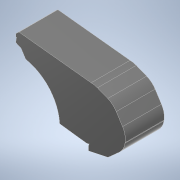
# Autodesk Inventor part: Pieza3_Carcasa
Saved by Autodesk Inventor 2022 (Build 260153000, 153)
## iProperties
Created: 2022-11-06
Part Number: Pieza3_Carcasa
Material: Resina acetálica, negra
Document SubType Name: Modeling
Designer: Mauricio Guerrero
Density: 1.425 g/cm^3
Appearance: Suave - Negro
Author: Mauricio Guerrero
## iProperties of the stored document Pieza3_Carcasa_3DPrint.ipt
Created: 2022-11-09
Part Number: Pieza3_Carcasa_3DPrint
Material: Genérico
Document SubType Name: Modeling
Designer: Mauricio Guerrero
Density: 1 g/cm^3
Appearance: Valor por defecto
Author: Mauricio Guerrero
Autodesk Inventor part; units mm, degrees
ref_plane "YZ Plane" through (0, 0, 0) normal (1, 0, 0) x (0, 1, 0)
ref_plane "XZ Plane" through (0, 0, 0) normal (0, 1, 0) x (-1, 0, 0)
ref_plane "XY Plane" through (0, 0, 0) normal (0, 0, 1) x (1, 0, 0)
sketch "Boceto1" plane through (0, 0, 0) normal (0, 0, 1) x (1, 0, 0)
  line L0 (8.9411, -4.2344) -> (11.6298, -3.6616)
  line L1 (11.6298, -3.6616) -> (13.3209, -2.1424)
  arc A0 (13.3209, -2.1424) -> (13.9587, -0.9739) centre (11.9843, -0.6546) ccw
  line L2 (13.9587, -0.9739) -> (13.978, -0.8543)
  arc A1 (9.9548, 3.6595) -> (9.2184, 3.8) centre (9.2184, 1.8) ccw
  line L3 (9.9548, 3.6595) -> (11.6833, 2.9749)
  arc A2 (12.6312, 2.1939) -> (11.6833, 2.9749) centre (10.9469, 1.1154) ccw
  line L4 (12.6312, 2.1939) -> (13.688, 0.5435)
  line L5 (14.1, 2.7373) -> (14.1, -1.982) construction
  arc A3 (13.978, -0.8543) -> (13.688, 0.5435) centre (12.0037, -0.535) ccw
  line L6 (-3.2, 5.1465) -> (9.2184, 3.8)
  arc A4 (10.323, 4.5892) -> (9.2779, 4.7994) centre (9.2184, 1.8) ccw
  line L7 (10.323, 4.5892) -> (12.0516, 3.9047)
  arc A5 (13.4734, 2.7331) -> (12.0516, 3.9047) centre (10.9469, 1.1154) ccw
  line L8 (13.4734, 2.7331) -> (14.5302, 1.0827)
  arc A6 (14.9652, -1.0139) -> (14.5302, 1.0827) centre (12.0037, -0.535) ccw
  line L9 (14.9652, -1.0139) -> (14.9459, -1.1335)
  arc A7 (13.9892, -2.8863) -> (14.9459, -1.1335) centre (11.9843, -0.6546) ccw
  line L10 (13.9892, -2.8863) -> (12.0994, -4.584)
  line L11 (12.0994, -4.584) -> (8.8118, -5.2844)
  line L12 (-2.782, 6.107) -> (9.2779, 4.7994)
  line L13 (9.2184, 3.8) -> (-3.2, 5.1465)
  line L14 (-3.2816, 5.1553) -> (-3.2, 5.1465)
  line L15 (8.8118, -4.6408) -> (8.9411, -4.2344)
  line L16 (-3.2816, 5.6583) -> (-2.782, 6.107)
  line L17 (-3.2816, 5.6583) -> (-3.2816, 5.1553)
  line L18 (8.8118, -5.2844) -> (8.8118, -4.6408)
  point P0 (0, 0)
  point P1 (14.1, -0.1)
  point P2 (9.6, 3.8)
  dimension "d1" = 2
  dimension "d2" = 1
  constraints: 38 end point, 16 point on circle, 8 centre point, 7 tangent, 4 point on line, 3 equal radius, 3 vertical, 1 collinear, 7 other
  measures "d1" radius of A2
  measures "d2" distance between parallel lines of L6 L12
extrude "Extrusión1" add sketch "Boceto1" along normal blind 6.5
sketch "Boceto2" plane through (0, 0, 6.5) normal (0, 0, 1) x (1, 0, 0)
  line L0 (7.1, -4.15) -> (7.1, -7.1226) construction
  line L1 (-3.2, 3.2) -> (-3.2, -3.4) construction
  line L2 (-1.4, 3.8) -> (-1.4, 6.2978) construction
  line L3 (14.1, 2.7373) -> (14.1, -1.982) construction
  line L4 (7.1, -4.15) -> (8.5447, -4.3189)
  line L5 (8.5447, -4.3189) -> (11.6298, -3.6616)
  line L6 (11.6298, -3.6616) -> (13.3209, -2.1424)
  line L7 (13.9587, -0.9739) -> (13.978, -0.8543)
  line L8 (9.9548, 3.6595) -> (11.6833, 2.9749)
  line L9 (12.6312, 2.1939) -> (13.688, 0.5435)
  arc A0 (12.6312, 2.1939) -> (11.6833, 2.9749) centre (10.9469, 1.1154) ccw
  arc A1 (9.9548, 3.6595) -> (9.2184, 3.8) centre (9.2184, 1.8) ccw
  arc A2 (13.978, -0.8543) -> (13.688, 0.5435) centre (12.0037, -0.535) ccw
  arc A3 (13.3209, -2.1424) -> (13.9587, -0.9739) centre (11.9843, -0.6546) ccw
  line L10 (-1.6574, 2.7373) -> (-2.4537, 3.981)
  line L11 (-2.4537, 3.981) -> (-3.3251, 4.3261)
  line L12 (-3.3251, 4.3261) -> (-3.2, 5.1465)
  line L13 (-3.2, 5.1465) -> (9.2184, 3.8)
  line L14 (7.1, -4.15) -> (4.0215, -3.7498)
  arc A4 (4.0215, -3.7498) -> (-1.6574, 2.7373) centre (-2.942, -4.1165) ccw
  point P0 (0, 0)
  point P1 (0, 0)
  point P2 (9.6, 3.8)
  point P3 (14.1, -0.1)
  dimension "d7" = 4.15
  dimension "d8" = 10.3
  dimension "d9" = 3.8
  dimension "d10" = 1.8
  dimension "d11" = 11
  dimension "d12" = 7
  dimension "d13" = 2
  constraints: 30 end point, 10 point on circle, 7 tangent, 5 centre point, 5 point on line, 4 vertical, 3 equal radius
  measures "d7" vertical distance of L4.start point (0, 0)
  measures "d8" distance between parallel lines of L0 L1
  measures "d9" vertical distance of point (0, 0) L2.start
  measures "d10" distance between parallel lines of L1 L2
  measures "d11" distance of L2.start point (9.6, 3.8)
  measures "d12" distance from line of L3 L4.start
  measures "d13" radius of A0
extrude "Extrusión2" add sketch "Boceto2" against normal blind 0.8
